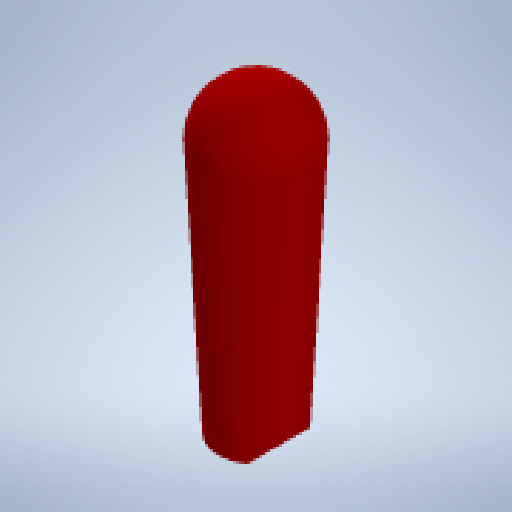
# Autodesk Inventor part: part4
Saved by Autodesk Inventor 2025.2 (Build 292293000, 293)
## iProperties
Created: 2024-12-08
Part Number: part4
Material: Kauczuk
Document SubType Name: Modeling
Designer: Marek
Density: 0.93 g/cm^3
Appearance: Kauczuk — czarny
Author: Marek
Autodesk Inventor part; units mm, degrees
ref_plane "YZ Plane" through (0, 0, 0) normal (1, 0, 0) x (0, 1, 0)
ref_plane "XZ Plane" through (0, 0, 0) normal (0, 1, 0) x (-1, 0, 0)
ref_plane "XY Plane" through (0, 0, 0) normal (0, 0, 1) x (1, 0, 0)
sketch "Szkic1" plane through (0, 0, 0) normal (0, 1, 0) x (-1, 0, 0)
  circle A0 centre (0, 0) radius 8.5
  dimension "d0" = 17
  constraints: 1 centre point, 1 coincident
  measures "d0" diameter of A0
extrude "Wyciągnięcie proste1" add sketch "Szkic1" along normal blind 57 draft 3
sketch "Szkic2" plane through (0, 57, 0) normal (0, 1, 0) x (1, 0, 0)
  circle A0 centre (0, 0) radius 11.4872
  line L0 (0, -11.4872) -> (0, 11.4872)
  constraints: 2 end point, 2 point on circle, 1 centre point, 1 coincident, 1 vertical
revolve "Obrót1" add sketch "Szkic2" angle 360 about axis through (0, 57, 11.4872) along (0, 0, -1) picked at (-4.984, 2.1752) contours L0 A0
sketch "Szkic3" plane through (0, 0, 0) normal (1, 0, 0) x (0, 1, 0)
  line L0 (0, 0) -> (0, -6.3)
  line L1 (0, -8.5) -> (0, 8.5) projected
  line L2 (55.7993, 11.4243) -> (55.7993, -11.4243) projected
  line L3 (0, 0) -> (0, 6.3)
  circle A0 centre (50, 0) radius 6.3
  line L4 (0, 6.3) -> (50, 6.3)
  line L5 (0, -6.3) -> (50, -6.3)
  point P0 (55.7993, 6.3)
  point P1 (50, 6.3)
  dimension "d4" = 6.3
  dimension "d5" = 6.3
  dimension "d13" = 50
  constraints: 8 end point, 3 point on line, 1 centre point, 1 horizontal, 1 perpendicular
  measures "d4" distance of L0.start L0.end
  measures "d5" distance of L0.start L3.end
  measures "d13" distance of L3.end L4.end
sketch "Szkic4" plane through (0, 0, 0) normal (0, 0, 1) x (1, 0, 0)
  line L0 (0, 0) -> (5, 0)
  line L1 (8.5, 0) -> (-8.5, 0) projected
  line L2 (5, 0) -> (10.8623, 5.8623)
  line L3 (10.8623, 5.8623) -> (10.8623, -4.5556)
  line L4 (0, 0) -> (-5, 0)
  line L5 (-5, 0) -> (-11.3925, 6.3925)
  line L6 (-11.3925, 6.3925) -> (-11.3925, -5.0943)
  line L7 (-11.3925, -5.0943) -> (10.8623, -5.0943)
  line L8 (10.8623, -5.0943) -> (10.8623, -4.5556)
  dimension "d8" = 5
  dimension "d9" = 135
  dimension "d10" = 5
  constraints: 16 end point, 4 perpendicular, 2 point on line
  measures "d8" distance of L0.start L0.end
  measures "d9" angle of L2 L0
  measures "d10" distance of L0.start L4.end
extrude "Wyciągnięcie proste3" cut sketch "Szkic4" along normal mid plane 30
extrude "Wyciągnięcie proste4" cut sketch "Szkic3" along normal mid plane 6
